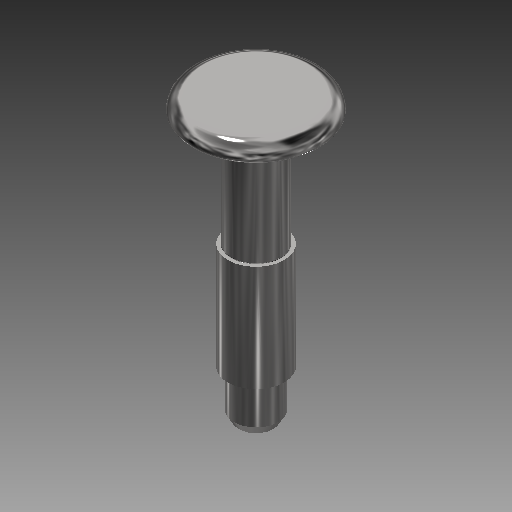
# Autodesk Inventor part: 100-02
Saved by Autodesk Inventor 2019 (Build 230136000, 136)
## iProperties
Company: Autodesk Inc.
Created: 2007-11-04
Part Number: 100-02
Document SubType Name: Modeling
Designer: Autodesk Inc.
Density: 8 g/cm^3
Mass: 17.1759 g
Surface Area: 14.5411 cm^2
Volume: 2.14699 cm^3
Material: Stainless Steel
Description: SPRING HOLDER PIN
Appearance: Steel - Polished
Component Category: Side Component
Author: Inventor
Autodesk Inventor part; units mm, degrees
ref_plane "YZ Plane" through (0, 0, 0) normal (1, 0, 0) x (0, 1, 0)
ref_plane "XZ Plane" through (0, 0, 0) normal (0, 1, 0) x (-1, 0, 0)
ref_plane "XY Plane" through (0, 0, 0) normal (0, 0, 1) x (1, 0, 0)
sketch "Sketch1" plane through (0, 0, 0) normal (0, 0, 1) x (1, 0, 0)
  line L0 (0, 0) -> (0, -38.8)
  line L1 (0, 0) -> (7, 0)
  line L2 (9, -2) -> (9, -2)
  line L3 (8.5, -2.5) -> (3.5, -2.5)
  line L4 (3.5, -2.5) -> (3.5, -18.5)
  line L5 (3.5, -18.5) -> (4, -18.5)
  line L6 (4, -18.5) -> (4, -33.5)
  line L7 (4, -33.5) -> (3.125, -33.5)
  line L8 (3.125, -33.5) -> (3.125, -38.8)
  line L9 (3.125, -38.8) -> (2.4322, -40)
  line L10 (2.4322, -40) -> (1.2738, -40)
  arc A0 (8.5, -2.5) -> (9, -2) centre (8.5, -2) ccw
  arc A1 (9, -2) -> (7, 0) centre (7, -2) ccw
  line L11 (0, -38.8) -> (1.2738, -40)
  dimension "d1" = 2.5
  dimension "d2" = 16
  dimension "d3" = 15
  dimension "d4" = 1.2
  dimension "d5" = 60
  dimension "d6" = 3.125
  dimension "d7" = 3.5
  dimension "d8" = 4
  dimension "d9" = 9
  dimension "d10" = 0.5
  dimension "d11" = 2
  dimension "d12" = 1.75
  dimension "d15" = 40
  constraints: 24 end point, 7 parallel, 4 point on circle, 4 tangent, 2 centre point, 2 perpendicular, 1 vertical
  measures "d1" distance between parallel lines of L1 L3
  measures "d2" distance of L3.end L4.end
  measures "d3" distance of L5.end L6.end
  measures "d4" distance from line of L8.end L10
  measures "d5" angle of L10 L9
  measures "d6" distance between parallel lines of L0 L8
  measures "d7" distance between parallel lines of L0 L4
  measures "d8" distance between parallel lines of L0 L6
  measures "d9" distance between parallel lines of L2 L0
  measures "d10" radius of A0
  measures "d11" radius of A1
  measures "d12" distance of L10.end L0.end
  measures "d15" distance between parallel lines of L1 L10
revolve "Revolution1" add sketch "Sketch1" angle 360 about axis through (0, 0, 0) along (0, -1, 0)
fillet "Fillet1" radius 0.1 2 edges at (-3.125, -33.5, 0) (-3.5, -18.5, 0)
fillet "Fillet2" radius 0.25 1 edges at (-3.5, -2.5, 0)
body "Solid1"
